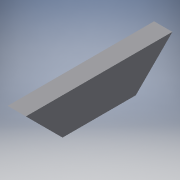
# Autodesk Inventor part: Arm Angle brace
Saved by Autodesk Inventor 2018.2 (Build 222227000, 227)
## iProperties
Created: 2018-02-08
Part Number: Arm Angle brace
Material: Generic
Document SubType Name: Modeling
Designer: jahu2
Density: 1 g/cm^3
Appearance: Default
Author: jahu2
Autodesk Inventor part; units mm, degrees
ref_plane "YZ Plane" through (0, 0, 0) normal (1, 0, 0) x (0, 1, 0)
ref_plane "XZ Plane" through (0, 0, 0) normal (0, 1, 0) x (-1, 0, 0)
ref_plane "XY Plane" through (0, 0, 0) normal (0, 0, 1) x (1, 0, 0)
sketch "Sketch1" plane through (0, 0, 0) normal (0, 0, 1) x (1, 0, 0)
  line L0 (0, 0) -> (-25.4, 0)
  line L1 (-25.4, 0) -> (-25.4, -50.8)
  line L2 (-25.4, -50.8) -> (0, -50.8)
  line L3 (0, -50.8) -> (0, 0)
  line L4 (-22.225, -3.175) -> (-3.175, -3.175)
  line L5 (-3.175, -3.175) -> (-3.175, -47.625)
  line L6 (-3.175, -47.625) -> (-22.225, -47.625)
  line L7 (-22.225, -47.625) -> (-22.225, -3.175)
  dimension "d0" = 25.4
  dimension "d1" = 50.8
  dimension "d2" = 3.175
  constraints: 16 end point, 4 parallel, 2 perpendicular, 1 horizontal, 3 other
  measures "d0" distance of L2.end L1.end
  measures "d1" distance of L1.end L0.end
  measures "d2" distance between parallel lines of L0 L4
extrude "Extrusion1" add sketch "Sketch1" along normal blind 203.2
sketch "Sketch2" plane through (0, -50.8, 0) normal (1, 0, 0) x (0, 0, -1)
  line L0 (-203.2, 50.8) -> (-152.4, 0)
  line L1 (0, 0) -> (-203.2, 0) projected
  line L2 (-203.2, 0) -> (-152.4, 0)
  line L3 (-203.2, 0) -> (-203.2, 50.8)
  line L4 (0, 50.8) -> (0, 0)
  line L5 (0, 50.8) -> (0, 0) projected
  line L6 (0, 0) -> (-50.8, 0)
  line L7 (0, 50.8) -> (-50.8, 0)
  dimension "d5" = 45
  dimension "d6" = 45
  dimension "d7" = 90
  dimension "d8" = 71.8421
  dimension "d9" = 50.8
  dimension "d10" = 50.8
  dimension "d11" = 45
  dimension "d12" = 45
  dimension "d13" = 71.8421
  constraints: 12 end point, 2 point on line, 1 collinear, 1 perpendicular, 1 vertical
  measures "d5" angle of L1 L0
  measures "d6" angle of L0 L3
  measures "d7" angle of L1 L3
  measures "d8" distance of L0.start L0.end
  measures "d9" distance of L1.end L0.start
  measures "d10" distance of L0.end L1.end
  measures "d11" angle of L1 L7
  measures "d12" angle of L4 L7
  measures "d13" distance of L4.start L6.end
extrude "Extrusion2" cut sketch "Sketch2" against normal blind 203.2
body "Solid1"
